Autodesk Inventor part; units mm, degrees
note: some values were not read from the file. Chosen so that the rebuilt part matches the saved one: sketch regions of "押し出し9".
(part 2 of 2)
sketch "スケッチ10" plane through (0, 0, 3) normal (0, 0, 1) x (1, 0, 0)
  circle A0 centre (70.4743, -10.4118) radius 1.5 projected
  circle A1 centre (138.2732, 5.5882) radius 2 projected
  circle A2 centre (80.4743, 23.124) radius 1.5 projected
  arc A3 (117.3199, -46.749) -> (137.4212, -31.9384) centre (110.4743, -16.4118) ccw projected
  line L0 (137.4212, -31.9384) -> (157.6055, 3.092) projected
  arc A4 (157.6055, 3.092) -> (156.8408, 9.0914) centre (153.2732, 5.5882) ccw projected
  line L1 (156.8408, 9.0914) -> (131.9243, 34.466) projected
  arc A5 (131.9243, 34.466) -> (126.5593, 36.1635) centre (127.6431, 30.2622) ccw projected
  line L2 (126.5593, 36.1635) -> (79.6614, 27.5499) projected
  arc A6 (79.6614, 27.5499) -> (76.162, 24.4099) centre (80.4743, 23.124) ccw projected
  line L3 (76.162, 24.4099) -> (66.162, -9.1259) projected
  arc A7 (66.162, -9.1259) -> (66.7172, -12.8885) centre (70.4743, -10.4118) ccw projected
  line L4 (66.7172, -12.8885) -> (90.988, -49.7066) projected
  arc A8 (90.988, -49.7066) -> (95.7356, -51.6195) centre (94.7451, -47.2298) ccw projected
  line L5 (95.7356, -51.6195) -> (117.3199, -46.749) projected
  line L6 (123.3635, 22.9728) -> (120.4296, 14.9968) projected
  arc A9 (118.0645, 13.7478) -> (120.4296, 14.9968) centre (118.5526, 15.6873) ccw projected
  arc A10 (118.0645, 13.7478) -> (106.6862, 14.4566) centre (110.4743, -16.4118) ccw projected
  arc A11 (104.4434, 16.5007) -> (106.6862, 14.4566) centre (106.4426, 16.4417) ccw projected
  arc A12 (104.4434, 16.5007) -> (96.7681, 14.1127) centre (100.1953, 16.6261) ccw projected
  arc A13 (96.0809, 11.157) -> (96.7681, 14.1127) centre (95.1553, 12.9299) ccw projected
  arc A14 (96.0809, 11.157) -> (94.4001, 10.212) centre (110.4743, -16.4118) ccw projected
  arc A15 (91.7731, 10.7152) -> (94.4001, 10.212) centre (93.3664, 11.9242) ccw projected
  line L7 (91.7731, 10.7152) -> (84.9801, 19.6674) projected
  arc A16 (84.6967, 21.568) -> (84.9801, 19.6674) centre (86.5734, 20.8764) ccw projected
  arc A17 (84.6967, 21.568) -> (84.9497, 23.594) centre (80.4743, 23.124) ccw projected
  arc A18 (86.5775, 25.77) -> (84.9497, 23.594) centre (86.9388, 23.8029) ccw projected
  line L8 (86.5775, 25.77) -> (118.2794, 31.5925) projected
  arc A19 (120.6357, 29.7665) -> (118.2794, 31.5925) centre (118.6406, 29.6254) ccw projected
  arc A20 (120.6357, 29.7665) -> (122.8508, 25.1256) centre (127.6431, 30.2622) ccw projected
  arc A21 (123.3635, 22.9728) -> (122.8508, 25.1256) centre (121.4865, 23.6632) ccw projected
  circle A22 centre (94.7451, -47.2298) radius 1.25 projected
  arc A23 (111.3601, -5.4224) -> (106.4151, -6.1613) centre (110.4743, -16.4118) ccw projected
  arc A24 (104.0855, -5.5107) -> (106.4151, -6.1613) centre (105.6787, -4.3018) ccw projected
  line L9 (104.0855, -5.5107) -> (96.0348, 5.0989) projected
  arc A25 (96.6437, 8.0488) -> (96.0348, 5.0989) centre (97.6281, 6.3079) ccw projected
  arc A26 (116.5511, 11.0233) -> (96.6437, 8.0488) centre (110.4743, -16.4118) ccw projected
  arc A27 (117.9957, 8.3801) -> (116.5511, 11.0233) centre (116.1186, 9.0706) ccw projected
  line L10 (117.9957, 8.3801) -> (113.3978, -4.1194) projected
  arc A28 (111.3601, -5.4224) -> (113.3978, -4.1194) centre (111.5208, -3.4289) ccw projected
  line L11 (116.2133, -5.1551) -> (120.8112, 7.3444) projected
  arc A29 (123.6242, 8.4215) -> (120.8112, 7.3444) centre (122.6883, 6.654) ccw projected
  arc A30 (133.5175, -0.33) -> (123.6242, 8.4215) centre (110.4743, -16.4118) ccw projected
  arc A31 (132.7917, -3.2534) -> (133.5175, -0.33) centre (131.8774, -1.4746) ccw projected
  line L12 (132.7917, -3.2534) -> (120.9467, -9.3421) projected
  arc A32 (118.5647, -8.922) -> (120.9467, -9.3421) centre (120.0323, -7.5633) ccw projected
  arc A33 (118.5647, -8.922) -> (116.9209, -7.468) centre (110.4743, -16.4118) ccw projected
  arc A34 (116.2133, -5.1551) -> (116.9209, -7.468) centre (118.0904, -5.8455) ccw projected
  arc A35 (101.695, -9.7429) -> (100.4118, -11.9067) centre (110.4743, -16.4118) ccw projected
  arc A36 (98.2897, -13.0673) -> (100.4118, -11.9067) centre (98.5864, -11.0895) ccw projected
  line L13 (98.2897, -13.0673) -> (85.1187, -11.0917) projected
  arc A37 (83.4952, -8.5546) -> (85.1187, -11.0917) centre (85.4154, -9.1138) ccw projected
  arc A38 (90.64, 3.4932) -> (83.4952, -8.5546) centre (110.4743, -16.4118) ccw projected
  arc A39 (93.645, 3.2855) -> (90.64, 3.4932) centre (92.0517, 2.0765) ccw projected
  line L14 (93.645, 3.2855) -> (101.6956, -7.3242) projected
  arc A40 (101.695, -9.7429) -> (101.6956, -7.3242) centre (100.1024, -8.5331) ccw projected
  circle A41 centre (100.1953, 16.6261) radius 1.25 projected
  circle A42 centre (144.4932, -10.0968) radius 1.25 projected
  arc A43 (74.5837, -8.578) -> (72.0881, -6.2111) centre (70.4743, -10.4118) ccw projected
  arc A44 (70.8888, -3.7727) -> (72.0881, -6.2111) centre (72.8054, -4.3442) ccw projected
  line L15 (70.8888, -3.7727) -> (77.185, 17.3421) projected
  arc A45 (79.524, 18.7255) -> (77.185, 17.3421) centre (79.1016, 16.7706) ccw projected
  arc A46 (79.524, 18.7255) -> (80.8362, 18.6385) centre (80.4743, 23.124) ccw projected
  arc A47 (82.5903, 17.854) -> (80.8362, 18.6385) centre (80.997, 16.645) ccw projected
  line L16 (82.5903, 17.854) -> (89.3833, 8.9018) projected
  arc A48 (89.1607, 6.2363) -> (89.3833, 8.9018) centre (87.79, 7.6928) ccw projected
  arc A49 (89.1607, 6.2363) -> (80.3787, -8.5721) centre (110.4743, -16.4118) ccw projected
  arc A50 (78.1466, -10.0459) -> (80.3787, -8.5721) centre (78.4432, -8.068) ccw projected
  line L17 (78.1466, -10.0459) -> (76.1135, -9.7409) projected
  arc A51 (74.5837, -8.578) -> (76.1135, -9.7409) centre (76.4101, -7.763) ccw projected
  line L18 (123.2452, 13.9611) -> (126.1791, 21.9371) projected
  arc A52 (127.9646, 23.2445) -> (126.1791, 21.9371) centre (128.0561, 21.2466) ccw projected
  arc A53 (127.9646, 23.2445) -> (133.0902, 25.8259) centre (127.6431, 30.2622) ccw projected
  arc A54 (136.068, 25.9642) -> (133.0902, 25.8259) centre (134.641, 24.563) ccw projected
  line L19 (136.068, 25.9642) -> (147.8266, 13.9895) projected
  arc A55 (146.3996, 10.5882) -> (147.8266, 13.9895) centre (146.3996, 12.5882) ccw projected
  line L20 (146.3996, 10.5882) -> (138.2732, 10.5882) projected
  arc A56 (138.2732, 10.5882) -> (133.802, 7.8261) centre (138.2732, 5.5882) ccw projected
  arc A57 (130.712, 7.2027) -> (133.802, 7.8261) centre (132.0135, 8.7213) ccw projected
  arc A58 (130.712, 7.2027) -> (124.2371, 11.4772) centre (110.4743, -16.4118) ccw projected
  arc A59 (123.2452, 13.9611) -> (124.2371, 11.4772) centre (125.1222, 13.2707) ccw projected
  line L21 (116.6595, -43.8226) -> (100.4182, -47.4874) projected
  arc A60 (99.2066, -46.6425) -> (100.4182, -47.4874) centre (100.1981, -46.512) ccw projected
  arc A61 (99.2066, -46.6425) -> (98.3892, -44.5896) centre (94.7451, -47.2298) ccw projected
  arc A62 (98.3083, -43.5483) -> (98.3892, -44.5896) centre (99.1989, -44.0029) ccw projected
  line L22 (98.3083, -43.5483) -> (106.107, -28.2683) projected
  arc A63 (108.2854, -27.2173) -> (106.107, -28.2683) centre (107.8884, -29.1775) ccw projected
  arc A64 (108.2854, -27.2173) -> (121.2735, -14.1917) centre (110.4743, -16.4118) ccw projected
  arc A65 (122.3182, -12.0102) -> (121.2735, -14.1917) centre (123.2325, -13.789) ccw projected
  line L23 (122.3182, -12.0102) -> (134.1632, -5.9215) projected
  arc A66 (136.9629, -7.0327) -> (134.1632, -5.9215) centre (135.0776, -7.7003) ccw projected
  arc A67 (116.6595, -43.8226) -> (136.9629, -7.0327) centre (110.4743, -16.4118) ccw projected
  line L24 (140.4335, -2.6984) -> (146.3968, 0.367) projected
  arc A68 (147.3112, 0.5882) -> (146.3968, 0.367) centre (147.3112, -1.4118) ccw projected
  line L25 (147.3112, 0.5882) -> (149.2398, 0.5882) projected
  arc A69 (150.9727, -2.4103) -> (149.2398, 0.5882) centre (149.2398, -1.4118) ccw projected
  line L26 (150.9727, -2.4103) -> (149.151, -5.572) projected
  arc A70 (146.4821, -6.341) -> (149.151, -5.572) centre (147.4181, -4.5735) ccw projected
  arc A71 (146.4821, -6.341) -> (142.4011, -6.3974) centre (144.4932, -10.0968) ccw projected
  arc A72 (139.547, -5.3668) -> (142.4011, -6.3974) centre (141.4166, -4.6565) ccw projected
  arc A73 (139.547, -5.3668) -> (139.4824, -5.1983) centre (110.4743, -16.4118) ccw projected
  arc A74 (140.4335, -2.6984) -> (139.4824, -5.1983) centre (141.3478, -4.4771) ccw projected
  arc A75 (78.7483, -25.6886) -> (80.5456, -24.8663) centre (79.5832, -25.1382) ccw projected
  line L27 (78.7483, -25.6886) -> (72.7888, -16.6482) projected
  arc A76 (73.2327, -13.9673) -> (72.7888, -16.6482) centre (74.4587, -15.5475) ccw projected
  arc A77 (73.2327, -13.9673) -> (73.8649, -13.3706) centre (70.4743, -10.4118) ccw projected
  arc A78 (75.6684, -12.7077) -> (73.8649, -13.3706) centre (75.3718, -14.6856) ccw projected
  line L28 (75.6684, -12.7077) -> (77.7015, -13.0127) projected
  arc A79 (79.403, -15.0764) -> (77.7015, -13.0127) centre (77.4049, -14.9905) ccw projected
  arc A80 (79.403, -15.0764) -> (80.5456, -24.8663) centre (110.4743, -16.4118) ccw projected
  circle A81 centre (127.6431, 30.2622) radius 4.025 projected
  circle A82 centre (153.2732, 5.5882) radius 2 projected
  circle A83 centre (110.4743, -16.4118) radius 10 projected
  line L29 (87.7126, -39.2018) -> (83.4326, -24.0508) projected
  arc A84 (82.3772, -16.0076) -> (83.4326, -24.0508) centre (110.4743, -16.4118) ccw projected
  arc A85 (84.6737, -14.0585) -> (82.3772, -16.0076) centre (84.377, -16.0364) ccw projected
  line L30 (84.6737, -14.0585) -> (97.8447, -16.0341) projected
  arc A86 (99.5329, -17.7663) -> (97.8447, -16.0341) centre (97.548, -18.012) ccw projected
  arc A87 (99.5329, -17.7663) -> (103.0079, -24.5237) centre (110.4743, -16.4118) ccw projected
  arc A88 (103.4349, -26.9045) -> (103.0079, -24.5237) centre (101.6535, -25.9953) ccw projected
  line L31 (103.4349, -26.9045) -> (95.6362, -42.1845) projected
  arc A89 (94.7454, -42.7298) -> (95.6362, -42.1845) centre (94.7455, -41.7298) ccw projected
  arc A90 (94.7454, -42.7298) -> (91.9371, -43.7135) centre (94.7451, -47.2298) ccw projected
  arc A91 (90.4782, -43.4824) -> (91.9371, -43.7135) centre (91.3131, -42.932) ccw projected
  line L32 (90.4782, -43.4824) -> (87.84, -39.4804) projected
  arc A92 (87.7126, -39.2018) -> (87.84, -39.4804) centre (88.6749, -38.93) ccw projected
  circle A93 centre (110.4743, -16.4118) radius 7.025 projected
  point P0 (0, 0)
